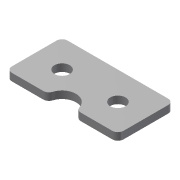
# Autodesk Inventor part: 30289-01
Saved by Autodesk Inventor 2014 (Build 180170000, 170)
## iProperties
Category: NS
Created: 2013-07-17
Part Number: 30289-01
Material: Steel, Mild
Document SubType Name: Modeling
Designer: Edward
Density: 7.86 g/cm^3
Appearance: Steel
Description: Z-Axis Shim Plate (12ga)
Project: Shapeoko
User Status: F
Vendor: ProkTech
Stock Number: S2Z2-01
Authority: PER BARRY PROCK 9-16-13
Author: Edward
Subject: Structural
Comments: Fusion
Title: Z Shim Plate
Autodesk Inventor part; units mm, degrees
ref_plane "YZ Plane" through (0, 0, 0) normal (1, 0, 0) x (0, 1, 0)
ref_plane "XZ Plane" through (0, 0, 0) normal (0, 1, 0) x (-1, 0, 0)
ref_plane "XY Plane" through (0, 0, 0) normal (0, 0, 1) x (1, 0, 0)
sketch "Sketch1" plane through (0, 0, 0) normal (0, 0, 1) x (1, 0, 0)
  line L0 (-20, 10) -> (20, 10)
  line L1 (20, 10) -> (20, -10)
  line L2 (-20, -10) -> (-20, 10)
  arc A0 (5, -10) -> (-5, -10) centre (0, -10) ccw
  line L3 (20, -10) -> (5, -10)
  line L4 (-5, -10) -> (-20, -10)
  point P0 (0, 0)
  dimension "d0" = 40
  dimension "d1" = 20
  dimension "d2" = 20
  dimension "d3" = 10
  dimension "d4" = 10
  dimension "d5" = 20
  dimension "d6" = 20
  dimension "d7" = 15
  constraints: 10 end point, 3 parallel, 2 point on circle, 1 centre point, 1 horizontal, 1 perpendicular
  measures "d0" distance of L1.end L2.start
  measures "d1" distance of L0.end L1.end
  measures "d2" distance from line of point (0, 0) L2
  measures "d3" distance from line of L0 point (0, 0)
  measures "d4" diameter of A0
  measures "d5" distance from line of L2 A0.centre
  measures "d6" distance from line of L0 A0.centre
  measures "d7" distance of L2.start L4.start
extrude "Extrusion1" add sketch "Sketch1" along normal blind 2.6568
sketch "Sketch2" plane through (0, 0, 2.6568) normal (0, 0, 1) x (1, 0, 0)
  line L0 (20, 10) -> (-20, 10) projected
  line L1 (-20, 10) -> (-20, -10) projected
  circle A0 centre (-10, 0) radius 2.75
  circle A1 centre (10, 0) radius 2.75
  point P0 (0, 0)
  dimension "d23" = 5.5
  dimension "d24" = 10
  dimension "d25" = 10
  dimension "d28" = 20
  constraints: 2 centre point, 1 horizontal, 2 other
  measures "d23" diameter of A0
  measures "d24" distance from line of L0 A0.centre
  measures "d25" distance from line of L1 A0.centre
  measures "d28" distance of A0.centre A1.centre
extrude "Extrusion2" cut sketch "Sketch2" against normal through all
fillet "Fillet1" radius 2 4 edges at (20, -10, 1.3284) (-20, -10, 1.3284) (-5, -10, 1.3284) (5, -10, 1.3284)
fillet "Fillet2" radius 2 2 edges at (20, 10, 1.3284) (-20, 10, 1.3284)
equation "\"d2\" = 0.5 * d0"
equation "\"d3\" = 0.5 * d1"
equation "\"d25\" = d24"
body "Solid1"
